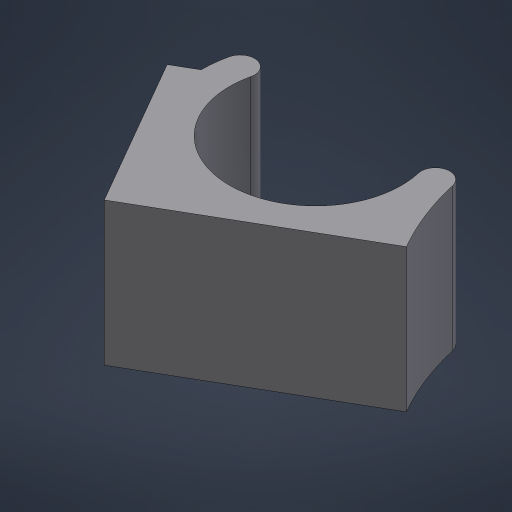
# Autodesk Inventor part: baztholder
Saved by Autodesk Inventor 2023.5 (Build 275446000, 446)
## iProperties
Created: 2025-03-21
Part Number: baztholder
Material: Generisch
Document SubType Name: Modeling
Designer: David Lill
Density: 1 g/cm^3
Appearance: Vorgabe
Author: David Lill
Autodesk Inventor part; units mm, degrees
ref_plane "YZ Plane" through (0, 0, 0) normal (1, 0, 0) x (0, 1, 0)
ref_plane "XZ Plane" through (0, 0, 0) normal (0, 1, 0) x (-1, 0, 0)
ref_plane "XY Plane" through (0, 0, 0) normal (0, 0, 1) x (1, 0, 0)
sketch "Skizze1" plane through (0, 0, 0) normal (0, 0, 1) x (1, 0, 0)
  circle A0 centre (0, 0) radius 9
  circle A1 centre (0, 0) radius 12
  arc A2 (-8.775, 2) -> (-11.7, 2.6667) centre (-10.2375, 2.3333) ccw
  arc A3 (11.7, 2.6667) -> (8.775, 2) centre (10.2375, 2.3333) ccw
  line L0 (-12, 0) -> (-14.2583, -1.3038)
  line L1 (-14.2583, -1.3038) -> (-5.2583, -16.8923)
  line L2 (-5.2583, -16.8923) -> (6, -10.3923)
  line L3 (0, -22.6708) -> (0, 17.7785) projected
  line L4 (6, -10.3923) -> (14.8243, -5.2976)
  arc A4 (11.7, 2.6667) -> (14.8243, -5.2976) centre (39.6544, 9.0381) ccw
  dimension "d0" = 18
  dimension "d1" = 3
  dimension "d2" = 2
  dimension "d4" = 18
  dimension "d5" = 13
  dimension "d6" = 120
  constraints: 12 point on circle, 8 end point, 7 tangent, 5 centre point, 2 perpendicular, 1 coincident, 1 horizontal alignment, 1 line through centre
  measures "d0" diameter of A0
  measures "d1" radial gap between concentric circles of A0 A1
  measures "d2" vertical distance of point (0, 0) A0.end
  measures "d4" distance from line of L1.end L0
  measures "d5" distance from line of point (0, 0) L1
  measures "d6" angle of L3 L2
extrude "Extrusion1" add sketch "Skizze1" along normal mid plane 15 contours A0 A3 A1 L3 | L3 A1 A2 A0 | A4 L4 A1 | L3 L2 L1 L0 A1 | A1 L2 L3 picked at (10.9126, -0.8316) picked at (-1.5575, -10.8245)
